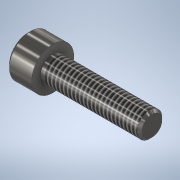
# Autodesk Inventor part: CBE5-20
Saved by Autodesk Inventor 2022 (Build 260153000, 153)
## iProperties
Category: PARTsolutions
Company: MISUMI
Created: 2022-12-14
Part Number: CBE5-20
Material: Generic
Catalog Web Link: www.cadenas.de
Description: CBE-Hexagon Socket Head Cap Screws -Trivalent Chromate-
Vendor: MISUMI
Document SubType Name: Modeling
Designer: psAdmin
Manufacturer: MISUMI
Mass: 0.631973 g
Surface Area: 5.84779 cm^2
Volume: 0.631973 cm^3
Density: 1 g/cm^3
Appearance: 鋼 - つや出し
PSOL_IDENT_0: {$CADENAS_DATA/23d-libs/misumi/metric/27_screws_nuts/cbe.prj},153 {VTYP=3D},{NB=CBE5-20},{LINA=CBE5-
PSOL_IDENT_1: 20},{NN=CBE},{DATE=31.05.2022 09:36:26},{GEOMDATE=29.01.2020 09:52:26},{VERSION=},{LINEID=80},{WBVAR=
PSOL_IDENT_2: L},{WBNUMERIC=L}  {NB=CBE5-20},{LINA=CBE5-20},{KT=DUMMY},{PN=CBE5-20},{TYPE=CBE},{M=5},{M1=5.0},{L=2
PSOL_IDENT_3: 0},{L0=6,8,10,12,15,18,20,25,30,35,40,45,50},{LL1=20},{LL=Full Thread},{P=0.80},{A=8.5},{E=5.0},{B=4
PSOL_IDENT_4: .0},{TT=2.5},{VV=0.50}
NB: CBE5-20
NN: CBE
NT: Hexagon Socket Head Cap Screws -Trivalent Chromate-
NBSYN: $PN.
LINA: CBE5-20
CATALOG: Misumi
PN: CBE5-20
M: 5
L: 20
LL: Full Thread
P: 0.8
A: 8.5
E: 5
B: 4
SUPPLIER: MISUMI
ARTICLENO: CBE5-20
BOMINFO: CBE5-20
CREATOR: CADENAS GmbH
Title: CBE5-20
Author: Cadenas PARTsolutions
Comments: Hexagon Socket Head Cap Screws -Trivalent Chromate-
Autodesk Inventor part; units mm, degrees
sketch "Sketch_1" plane through (0, 0, 0) normal (0, 0, 1) x (1, 0, 0)
  line L0 (20, 0) -> (-5, 0)
  line L1 (-5, 0) -> (-5, 3.75)
  line L2 (-5, 3.75) -> (-4.5, 4.25)
  line L3 (-4.5, 4.25) -> (0, 4.25)
  line L4 (0, 4.25) -> (0, 2.5)
  line L5 (0, 2.5) -> (19.5095, 2.5)
  line L6 (19.5095, 2.5) -> (20, 2.0095)
  line L7 (20, 2.0095) -> (20, 0)
  line L8 (20, 0) -> (-5, 0)
  constraints: 18 end point
revolve "Revolution1" add sketch "Sketch_1" angle 360 about axis through (20, 0, 0) along (1, 0, 0)
thread "Thread1" size "M5x0.8" class "6g" standard "ISO Metric profile" length 19.2 offset 0.8
sketch "Sketch2" plane through (-5, 0, 0) normal (-1, 0, 0) x (0, 0, 1)
  point P0 (0, 0)
hole "Hole1" at (-5, 0, 0) direction (1, 0, 0) diameter 4 depth 2.5 tip angle 120
sketch "Sketch_3" plane through (-5, 0, 0) normal (1, 0, 0) x (0, 0, -1)
  line L0 (-2, -1.1547) -> (0, -2.3094)
  line L1 (0, -2.3094) -> (2, -1.1547)
  line L2 (2, -1.1547) -> (2, 1.1547)
  line L3 (2, 1.1547) -> (0, 2.3094)
  line L4 (0, 2.3094) -> (-2, 1.1547)
  line L5 (-2, 1.1547) -> (-2, -1.1547)
  constraints: 12 end point
extrude "Extrusion1" cut sketch "Sketch_3" along normal blind 2.5
ref_plane "bolt_XY" through (20, 0, 0) normal (1, 0, 0) x (0, 0, -1)
ref_plane "bolt_YZ" through (20, 0, 0) normal (0, 0, -1) x (0, 1, 0)
ref_plane "bolt_ZX" through (20, 0, 0) normal (0, 1, 0) x (1, 0, 0)
ref_plane "nut_XY" through (0, 0, 0) normal (1, 0, 0) x (0, 0, -1)
ref_plane "nut_YZ" through (0, 0, 0) normal (0, 0, -1) x (0, 1, 0)
ref_plane "nut_ZX" through (0, 0, 0) normal (0, 1, 0) x (1, 0, 0)
body "Solid1"
